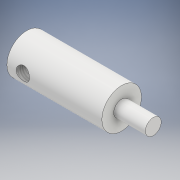
# Autodesk Inventor part: brazos_planetarios1
Saved by Autodesk Inventor 2018 (Build 220112000, 112)
## iProperties
Created: 2019-06-24
Part Number: brazos_planetarios1
Material: Nilón 6/6
Document SubType Name: Modeling
Designer: Cristiano
Density: 1.13 g/cm^3
Appearance: Blanco
Author: Cristiano
Autodesk Inventor part; units mm, degrees
ref_plane "YZ Plane" through (0, 0, 0) normal (1, 0, 0) x (0, 1, 0)
ref_plane "XZ Plane" through (0, 0, 0) normal (0, 1, 0) x (-1, 0, 0)
ref_plane "XY Plane" through (0, 0, 0) normal (0, 0, 1) x (1, 0, 0)
sketch "Boceto3" plane through (0, 0, 0) normal (0, 0, 1) x (1, 0, 0)
  line L0 (0, 0) -> (0, 12.5)
  line L1 (0, 12.5) -> (60, 12.5)
  line L2 (60, 12.5) -> (60, 5)
  line L3 (60, 5) -> (80, 5)
  line L4 (80, 5) -> (80, 0)
  line L5 (80, 0) -> (0, 0)
  dimension "d16" = 12.5
  dimension "d17" = 60
  dimension "d18" = 20
  dimension "d19" = 5
  constraints: 12 end point, 5 perpendicular, 1 vertical
  measures "d16" distance of L0.start L0.end
  measures "d17" distance of L0.end L1.end
  measures "d18" distance of L2.end L3.end
  measures "d19" distance of L3.end L4.end
revolve "Revolución1" add sketch "Boceto3" angle 360 about axis through (80, 0, 0) along (-1, 0, 0)
sketch "Boceto4" plane through (0, 0, 0) normal (0, 1, 0) x (-1, 0, 0)
  circle A0 centre (-10, 0) radius 4.25
  line L0 (-60, 12.5) -> (-60, -12.5) projected
  point P0 (0, 0)
  dimension "d21" = 8.5
  dimension "d22" = 50
  constraints: 1 centre point
  measures "d21" diameter of A0
  measures "d22" distance from line of L0 A0.centre
extrude "Extrusión3" cut sketch "Boceto4" along normal through all both and the other way through all
thread "Rosca3" size "M10x1.5" class "6H" standard "ANSI Metric M Profile" full length
thread "Rosca4" size "M10x1.5" class "6g" standard "ANSI Metric M Profile" full length
